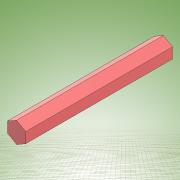
# Autodesk Inventor part: Eje
Saved by Autodesk Inventor 2022 (Build 260153000, 153)
## iProperties
Created: 2022-03-05
Part Number: Eje
Material: Genérico
Document SubType Name: Modeling
Designer: Marco
Density: 1 g/cm^3
Appearance: Valor por defecto
Author: Marco
Autodesk Inventor part; units mm, degrees
ref_plane "YZ Plane" through (0, 0, 0) normal (1, 0, 0) x (0, 1, 0)
ref_plane "XZ Plane" through (0, 0, 0) normal (0, 1, 0) x (-1, 0, 0)
ref_plane "XY Plane" through (0, 0, 0) normal (0, 0, 1) x (1, 0, 0)
sketch "Boceto1" plane through (0, 0, 0) normal (0, 0, 1) x (1, 0, 0)
  line L0 (0, 3.2332) -> (2.8, 1.6166)
  line L1 (2.8, 1.6166) -> (2.8, -1.6166)
  line L2 (2.8, -1.6166) -> (0, -3.2332)
  line L3 (0, -3.2332) -> (-2.8, -1.6166)
  line L4 (-2.8, -1.6166) -> (-2.8, 1.6166)
  line L5 (-2.8, 1.6166) -> (0, 3.2332)
  point P0 (0, 0)
  point P1 (0, 0)
  point P2 (2.8, 0)
  dimension "d0" = 5.6
  constraints: 12 end point, 1 coincident, 1 horizontal alignment, 1 midpoint, 13 other
  measures "d0" distance of L1.end L3.end
extrude "Extrusión1" add sketch "Boceto1" along normal blind 45
